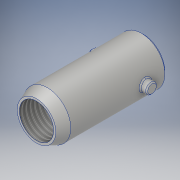
# Autodesk Inventor part: support_douille
Saved by Autodesk Inventor 2019 (Build 230136000, 136)
## iProperties
Created: 2019-03-25
Part Number: support_douille
Material: Aluminium 6061
Document SubType Name: Modeling
Designer: theor
Density: 2.7 g/cm^3
Appearance: Aluminium - Plat
Mass: 25.5705 g
Surface Area: 61.9904 cm^2
Volume: 9.47055 cm^3
Author: theor
Autodesk Inventor part; units mm, degrees
ref_plane "XZ Plane" through (0, 0, 0) normal (0, 1, 0) x (-1, 0, 0)
ref_plane "XY Plane" through (0, 0, 0) normal (0, 0, 1) x (1, 0, 0)
sketch "Esquisse1" plane through (0, 0, 0) normal (1, 0, 0) x (0, 1, 0)
  line L0 (0, 0) -> (0, 17.1522)
  line L1 (8, 50) -> (8, 36)
  line L2 (8, 36) -> (6, 36)
  line L3 (6, 36) -> (6, 30)
  line L4 (6, 30) -> (8, 24.505)
  line L5 (8, 24.505) -> (8, 1)
  line L6 (8, 1) -> (9, 0)
  line L7 (9, 0) -> (10, 0)
  line L8 (8, 50) -> (9, 50)
  line L9 (9, 50) -> (11, 45)
  line L10 (11, 45) -> (11, 1)
  line L11 (11, 1) -> (10, 0)
  dimension "d0" = 160
  dimension "d1" = 6
  dimension "d2" = 14
  dimension "d4" = 16
  dimension "d6" = 16
  dimension "d8" = 1
  dimension "d9" = 1
  dimension "d10" = 30
  dimension "d11" = 1
  dimension "d12" = 2
  dimension "d13" = 22
  dimension "d14" = 3
  dimension "d15" = 5
  dimension "d19" = 1
  dimension "d20" = 1
  constraints: 25 end point, 5 vertical, 3 horizontal, 1 horizontal alignment
  measures "d0" angle of L3 L4
  measures "d1" distance of L2.end L3.end
  measures "d2" distance of L1.start L1.end
  measures "d4" diameter of L1 L0
  measures "d6" diameter of L5 L0
  measures "d8" horizontal distance of L5.end L6.end
  measures "d9" horizontal distance of L5.end L6.end
  measures "d10" vertical distance of L3.end L6.end
  measures "d11" distance of L1.start L8.end
  measures "d12" distance between parallel lines of L3 L1
  measures "d13" diameter of L10 L0
  measures "d14" distance between parallel lines of L10 L5
  measures "d15" vertical distance of L8.end L9.end
  measures "d19" horizontal distance of L10.end L7.end
  measures "d20" horizontal distance of L10.end L7.end
revolve "Révolution1" add sketch "Esquisse1" angle 360 about axis through (0, 0, 0) along (0, 0, 1)
thread "Filetage1" size "M16x2" class "6H" standard "ISO Metric profile" full length
ref_plane "Plan de construction2" through (14, 0, 0) normal (1, 0, 0) x (0, 1, 0)
sketch "Esquisse2" plane through (14, 0, 0) normal (1, 0, 0) x (0, 1, 0)
  circle A0 centre (0, 10) radius 2.5
  point P0 (0, 0)
  dimension "d22" = 5
  dimension "d23" = 10
  constraints: 1 centre point, 1 vertical alignment
  measures "d22" diameter of A0
  measures "d23" distance of A0.centre point (0, 0)
extrude "Extrusion1" add sketch "Esquisse2" against normal up to surface round surface about axis through (0, 0, 23) along (0, 0, -1) radius 11 far side no
chamfer "Chanfrein1" distance 0.5 angle 45 2 edges at (10.7122, -2.4999, 9.9778) (14, -2.5, 10)
pattern_circular "Réseau circulaire1" count 2 over 360 about axis through (0, 0, -10) along (0, 0, 1) of "Extrusion1", "Chanfrein1"
